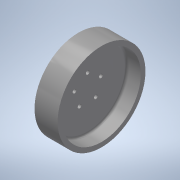
# Autodesk Inventor part: Interior_Rueda
Saved by Autodesk Inventor 2022.1 (Build 261234000, 234)
## iProperties
Created: 2021-09-22
Part Number: Interior_Rueda
Material: Genérico
Document SubType Name: Modeling
Designer: seb_0
Density: 1 g/cm^3
Appearance: Acero
Author: seb_0
Autodesk Inventor part; units mm, degrees
ref_plane "YZ Plane" through (0, 0, 0) normal (1, 0, 0) x (0, 1, 0)
ref_plane "XZ Plane" through (0, 0, 0) normal (0, 1, 0) x (-1, 0, 0)
ref_plane "XY Plane" through (0, 0, 0) normal (0, 0, 1) x (1, 0, 0)
sketch "Boceto1" plane through (0, 0, 0) normal (1, 0, 0) x (0, 1, 0)
  circle A0 centre (0, 0) radius 95
  circle A1 centre (0, 0) radius 85
  dimension "d0" = 190
  dimension "d1" = 170
  constraints: 2 centre point, 2 coincident
  measures "d0" diameter of A0
  measures "d1" diameter of A1
extrude "Extrusión1" add sketch "Boceto1" along normal blind 50
sketch "Boceto4" plane through (0, 0, 0) normal (-1, 0, 0) x (0, 0, 1)
  circle A0 centre (0, 0) radius 85 projected
  circle A1 centre (0, 0) radius 30
  circle A2 centre (0, 30) radius 4
  circle A3 centre (17.6336, -24.2705) radius 4
  circle A4 centre (-17.6336, -24.2705) radius 4
  circle A5 centre (-28.5317, 9.2705) radius 4
  circle A6 centre (28.5317, 9.2705) radius 4
  line L0 (0, 0) -> (0, 30)
  line L1 (0, 0) -> (28.5317, 9.2705)
  line L2 (0, 0) -> (-28.5317, 9.2705)
  line L3 (0, 0) -> (-17.6336, -24.2705)
  line L4 (0, 0) -> (17.6336, -24.2705)
  dimension "d5" = 60
  dimension "d6" = 8
  dimension "d7" = 8
  dimension "d8" = 8
  dimension "d9" = 8
  dimension "d10" = 8
  dimension "d11" = 72
  dimension "d12" = 72
  dimension "d13" = 72
  dimension "d14" = 72
  constraints: 10 end point, 6 centre point, 5 point on circle, 1 coincident, 1 vertical
  measures "d5" diameter of A1
  measures "d6" diameter of A2
  measures "d7" diameter of A3
  measures "d8" diameter of A4
  measures "d9" diameter of A5
  measures "d10" diameter of A6
  measures "d11" angle of L1 L0
  measures "d12" angle of L4 L1
  measures "d13" angle of L3 L4
  measures "d14" angle of L2 L3
extrude "Extrusión2" add sketch "Boceto4" against normal blind 20 contours A0 | A1 A3 L4 L1 A6 | L1 L0 A2 A1 A6 | A3 A1 A4 L3 L4 | L2 A5 A1 A2 L0 | L3 A4 A1 A5 L2
fillet "Empalme1" radius 5 1 edges at (20, -85, 0)
